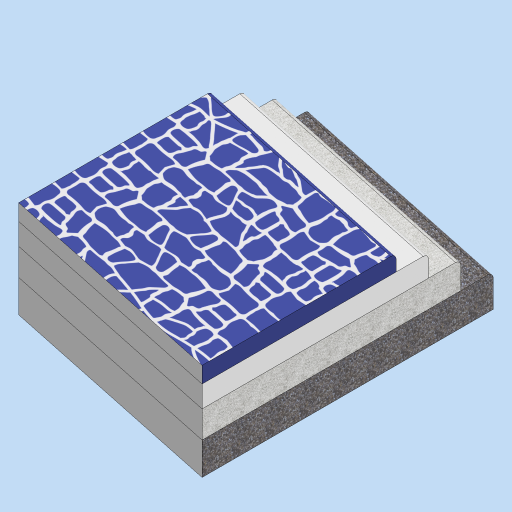
# Autodesk Inventor part: 콘크리트 제품 사진
Saved by Autodesk Inventor 2024.1 (Build 281209000, 209)
## iProperties
Created: 2024-01-18
Part Number: 콘크리트 제품 사진
Material: 일반
Document SubType Name: Modeling
Designer: KBU
Density: 1 g/cm^3
Appearance: 기본값
Author: KBU
Autodesk Inventor part; units mm, degrees
ref_plane "YZ Plane" through (0, 0, 0) normal (1, 0, 0) x (0, 1, 0)
ref_plane "XZ Plane" through (0, 0, 0) normal (0, 1, 0) x (-1, 0, 0)
ref_plane "XY Plane" through (0, 0, 0) normal (0, 0, 1) x (1, 0, 0)
sketch "스케치12" plane through (0, 0, 0) normal (0, 0, 1) x (1, 0, 0)
  line L0 (0, 0) -> (0, 450)
  line L1 (0, 450) -> (-850, 677.7568)
  line L2 (-850, 677.7568) -> (-850, 227.7568)
  line L3 (-850, 227.7568) -> (0, 0)
  line L4 (-257.118, 0) -> (130.0485, 0)
  line L5 (-850, 377.7568) -> (0, 150)
  line L6 (0, 275) -> (-850, 502.7568)
  line L7 (-850, 602.7568) -> (0, 375)
  dimension "d41" = 15
  dimension "d42" = 15
  dimension "d43" = 450
  dimension "d44" = 150
  dimension "d45" = 125
  dimension "d46" = 100
  dimension "d56" = 850
  constraints: 16 end point, 6 point on line, 5 parallel, 2 horizontal, 1 vertical
  measures "d41" angle of L3 L4
  measures "d42" angle of L4 L1
  measures "d43" distance of L1.end L2.end
  measures "d44" distance of L2.end L5.start
  measures "d45" distance of L5.start L6.end
  measures "d46" distance of L6.end L7.start
  measures "d56" distance between parallel lines of L0 L2
extrude "돌출12" add sketch "스케치12" against normal blind 1350 contours L3 L2 L5 L0
extrude "돌출13" add sketch "스케치12" against normal blind 1200 separate body contours L5 L2 L6 L0
extrude "돌출14" add sketch "스케치12" against normal blind 1050 separate body contours L6 L2 L7 L0
extrude "돌출15" add sketch "스케치12" against normal blind 900 separate body contours L7 L2 L1 L0
fillet "모깎기6" radius 25 4 edges at (-425, 263.8784, -1350) (-425, 388.8784, -1200) (-425, 488.8784, -1050) (-425, 563.8784, -900)
